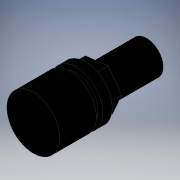
# Autodesk Inventor part: HTC-30M_5x20mmFuse_Holder
Saved by Autodesk Inventor 2016 (Build 200138000, 138)
## iProperties
Created: 2016-09-24
Part Number: HTC-30M_5x20mmFuse_Holder
Material: Generic
Document SubType Name: Modeling
Designer: jfixelle
Density: 1 g/cm^3
Appearance: Black
Author: jfixelle
Autodesk Inventor part; units mm, degrees
ref_plane "YZ Plane" through (0, 0, 0) normal (1, 0, 0) x (0, 1, 0)
ref_plane "XZ Plane" through (0, 0, 0) normal (0, 1, 0) x (-1, 0, 0)
ref_plane "XY Plane" through (0, 0, 0) normal (0, 0, 1) x (1, 0, 0)
sketch "Sketch1" plane through (0, 0, 0) normal (0, 0, 1) x (1, 0, 0)
  circle A0 centre (0, 0) radius 8
  dimension "d0" = 16
  constraints: 1 centre point, 1 coincident
  measures "d0" diameter of A0
extrude "Extrusion1" add sketch "Sketch1" along normal blind 11
sketch "Sketch2" plane through (0, 0, 0) normal (0, 0, -1) x (-1, 0, 0)
  circle A0 centre (0, 0) radius 6.5
  dimension "d3" = 13
  constraints: 1 centre point, 1 coincident
  measures "d3" diameter of A0
extrude "Extrusion2" add sketch "Sketch2" along normal blind 2
sketch "Sketch3" plane through (0, 0, -2) normal (0, 0, -1) x (-1, 0, 0)
  circle A0 centre (0, 0) radius 8
  dimension "d6" = 16
  constraints: 1 centre point, 1 coincident
  measures "d6" diameter of A0
extrude "Extrusion3" add sketch "Sketch3" along normal blind 2.8
sketch "Sketch4" plane through (0, 0, -4.8) normal (0, 0, -1) x (-1, 0, 0)
  line L0 (-2.7723, 6.3494) -> (4.1126, 5.5756)
  line L1 (4.1126, 5.5756) -> (6.8849, -0.7738)
  line L2 (6.8849, -0.7738) -> (2.7723, -6.3494)
  line L3 (2.7723, -6.3494) -> (-4.1126, -5.5756)
  line L4 (-4.1126, -5.5756) -> (-6.8849, 0.7738)
  line L5 (-6.8849, 0.7738) -> (-2.7723, 6.3494)
  point P0 (0, 0)
  point P1 (0, 0)
  dimension "d9" = 6
  constraints: 12 end point, 1 coincident, 13 other
  measures "d9" distance from line of L5 point (0, 0)
extrude "Extrusion4" add sketch "Sketch4" along normal blind 4
sketch "Sketch5" plane through (0, 0, -8.8) normal (0, 0, -1) x (-1, 0, 0)
  circle A0 centre (0, 0) radius 5
  dimension "d12" = 10
  constraints: 1 centre point, 1 coincident
  measures "d12" diameter of A0
extrude "Extrusion5" add sketch "Sketch5" along normal blind 14.4
body "Solid1"
